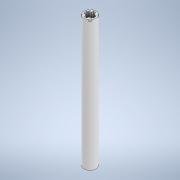
# Autodesk Inventor part: Upper Arm
Saved by Autodesk Inventor 2022 (Build 260153000, 153)
## iProperties
Created: 2022-03-03
Part Number: Upper Arm
Material: PLA Plastic
Document SubType Name: Modeling
Designer: Dahway
Density: 1.24912 g/cm^3
Appearance: PLA
Author: Dahway
Autodesk Inventor part; units mm, degrees
ref_plane "YZ Plane" through (0, 0, 0) normal (1, 0, 0) x (0, 1, 0)
ref_plane "XZ Plane" through (0, 0, 0) normal (0, 1, 0) x (-1, 0, 0)
ref_plane "XY Plane" through (0, 0, 0) normal (0, 0, 1) x (1, 0, 0)
sketch "Sketch1" plane through (0, 0, 0) normal (0, 1, 0) x (-1, 0, 0)
  circle A0 centre (0, 0) radius 7
  dimension "d0" = 14
  constraints: 1 centre point, 1 coincident
  measures "d0" diameter of A0
extrude "Extrusion1" add sketch "Sketch1" along normal blind 158
sketch "Sketch2" plane through (0, 158, 0) normal (0, 1, 0) x (1, 0, 0)
  circle A0 centre (0, 0) radius 3.75
  line L0 (-5.25, -1.5) -> (-2.25, -1.5)
  line L1 (-2.25, -1.5) -> (-2.25, 1.5)
  line L2 (-2.25, 1.5) -> (-5.25, 1.5)
  line L3 (-5.25, 1.5) -> (-5.25, -1.5)
  line L4 (-5.25, -1.5) -> (-2.25, 1.5) construction
  line L5 (-2.25, -1.5) -> (-5.25, 1.5) construction
  line L6 (-1.5, 2.25) -> (1.5, 2.25)
  line L7 (1.5, 2.25) -> (1.5, 5.25)
  line L8 (1.5, 5.25) -> (-1.5, 5.25)
  line L9 (-1.5, 5.25) -> (-1.5, 2.25)
  line L10 (-1.5, 2.25) -> (1.5, 5.25) construction
  line L11 (1.5, 2.25) -> (-1.5, 5.25) construction
  line L12 (2.25, 1.5) -> (5.25, 1.5)
  line L13 (5.25, 1.5) -> (5.25, -1.5)
  line L14 (5.25, -1.5) -> (2.25, -1.5)
  line L15 (2.25, -1.5) -> (2.25, 1.5)
  line L16 (2.25, 1.5) -> (5.25, -1.5) construction
  line L17 (5.25, 1.5) -> (2.25, -1.5) construction
  line L18 (-1.5, -5.25) -> (1.5, -5.25)
  line L19 (1.5, -5.25) -> (1.5, -2.25)
  line L20 (1.5, -2.25) -> (-1.5, -2.25)
  line L21 (-1.5, -2.25) -> (-1.5, -5.25)
  line L22 (-1.5, -5.25) -> (1.5, -2.25) construction
  line L23 (1.5, -5.25) -> (-1.5, -2.25) construction
  point P0 (-3.75, 0)
  point P1 (0, 3.75)
  point P2 (3.75, 0)
  point P3 (0, -3.75)
  point P4 (-3.4369, -1.5)
  point P5 (-1.5, -3.4369)
  point P6 (1.5, -3.4369)
  point P7 (3.4369, -1.5)
  point P8 (3.4369, 1.5)
  point P9 (1.5, 3.4369)
  point P10 (-1.5, 3.4369)
  point P11 (-3.4369, 1.5)
  dimension "d58" = 7.5
  dimension "d59" = 3
  dimension "d60" = 3
  dimension "d61" = 3
  dimension "d62" = 3
  dimension "d63" = 3
  dimension "d64" = 3
  dimension "d65" = 3
  dimension "d66" = 3
  constraints: 48 end point, 8 midpoint, 8 parallel, 4 horizontal, 4 perpendicular, 4 point on circle, 3 point on line, 1 centre point
  measures "d58" diameter of A0
  measures "d59" distance of L2.end L1.end
  measures "d60" distance of L1.end L0.end
  measures "d61" distance of L8.end L7.end
  measures "d62" distance of L7.end L6.end
  measures "d63" distance of L13.end L14.end
  measures "d64" distance of L12.end L13.end
  measures "d65" distance of L20.end L19.end
  measures "d66" distance of L19.end L18.end
extrude "Extrusion2" cut sketch "Sketch2" against normal through all
sketch "Sketch3" plane through (0, 158, 0) normal (0, 1, 0) x (1, 0, 0)
  circle A0 centre (0, 0) radius 9
  line L0 (-0.258, -9) -> (-0.258, -9)
  line L1 (-0.258, -11) -> (-0.258, -11)
  line L2 (-0.5, -9.5) -> (0.5, -9.5)
  line L3 (0.5, -9.5) -> (0.5, -8.5)
  line L4 (0.5, -8.5) -> (-0.5, -8.5)
  line L5 (-0.5, -8.5) -> (-0.5, -9.5)
  line L6 (-0.5, -9.5) -> (0.5, -8.5) construction
  line L7 (0.5, -9.5) -> (-0.5, -8.5) construction
  line L8 (-0.5, 8.5) -> (0.5, 8.5)
  line L9 (0.5, 8.5) -> (0.5, 9.5)
  line L10 (0.5, 9.5) -> (-0.5, 9.5)
  line L11 (-0.5, 9.5) -> (-0.5, 8.5)
  line L12 (-0.5, 8.5) -> (0.5, 9.5) construction
  line L13 (0.5, 8.5) -> (-0.5, 9.5) construction
  point P0 (0.492, 8.9865)
  point P1 (-0.258, -8.9963)
  point P2 (0, -9)
  point P3 (0, 9)
  point P4 (0.5, -8.9861)
  point P5 (-0.5, -8.9861)
  point P6 (-0.5, 8.9861)
  point P7 (0.5, 8.9861)
  dimension "d15" = 18
  dimension "d19" = 9
  dimension "d36" = 1
  dimension "d37" = 1
  dimension "d38" = 1
  dimension "d39" = 1
  constraints: 28 end point, 5 parallel, 4 midpoint, 4 point on circle, 3 horizontal, 2 perpendicular, 1 centre point, 1 coincident
  measures "d15" diameter of A0
  measures "d19" distance from line of A0.centre L0
  measures "d36" distance of L4.end L3.end
  measures "d37" distance of L3.end L2.end
  measures "d38" distance of L10.end L9.end
  measures "d39" distance of L9.end L8.end
extrude "Extrusion3" cut sketch "Sketch3" against normal blind 8
sketch "Sketch5" plane through (0, 0, 0) normal (0, -1, 0) x (1, 0, 0)
  line L0 (-1.25, 3.25) -> (-1.25, 1.25)
  line L1 (-1.25, 1.25) -> (-3.25, 1.25)
  line L2 (3.25, 1.25) -> (1.25, 1.25)
  line L3 (1.25, 1.25) -> (1.25, 3.25)
  line L4 (1.25, -3.25) -> (1.25, -1.25)
  line L5 (1.25, -1.25) -> (3.25, -1.25)
  line L6 (-3.25, -1.25) -> (-1.25, -1.25)
  line L7 (-1.25, -1.25) -> (-1.25, -3.25)
  circle A0 centre (0, 0) radius 3.75
  line L8 (-3.4369, -1.5) -> (-5.25, -1.5) projected
  line L9 (-2.25, 1.5) -> (-5.25, 1.5)
  line L10 (-5.25, 1.5) -> (-5.25, -1.5)
  line L11 (-5.25, -1.5) -> (-2.25, -1.5)
  line L12 (-2.25, -1.5) -> (-2.25, 1.5)
  line L13 (-2.25, 1.5) -> (-5.25, -1.5) construction
  line L14 (-5.25, 1.5) -> (-2.25, -1.5) construction
  line L15 (-1.5, -5.25) -> (-1.5, -3.4369) projected
  line L16 (1.5, -2.25) -> (-1.5, -2.25)
  line L17 (-1.5, -2.25) -> (-1.5, -5.25)
  line L18 (-1.5, -5.25) -> (1.5, -5.25)
  line L19 (1.5, -5.25) -> (1.5, -2.25)
  line L20 (1.5, -2.25) -> (-1.5, -5.25) construction
  line L21 (-1.5, -2.25) -> (1.5, -5.25) construction
  line L22 (1.5, 2.25) -> (-1.5, 2.25)
  line L23 (-1.5, 2.25) -> (-1.5, 5.25)
  line L24 (-1.5, 5.25) -> (1.5, 5.25)
  line L25 (1.5, 5.25) -> (1.5, 2.25)
  line L26 (1.5, 2.25) -> (-1.5, 5.25) construction
  line L27 (-1.5, 2.25) -> (1.5, 5.25) construction
  line L28 (5.25, 1.5) -> (5.25, -1.5) projected
  line L29 (2.25, 1.5) -> (5.25, 1.5)
  line L30 (5.25, 1.5) -> (5.25, -1.5)
  line L31 (5.25, -1.5) -> (2.25, -1.5)
  line L32 (2.25, -1.5) -> (2.25, 1.5)
  line L33 (2.25, 1.5) -> (5.25, -1.5) construction
  line L34 (5.25, 1.5) -> (2.25, -1.5) construction
  point P0 (-3.25, 3.25)
  point P1 (3.25, -3.25)
  point P2 (-3.75, 0)
  point P3 (0, -3.75)
  point P4 (0, 3.75)
  point P5 (3.75, 0)
  point P6 (3.4369, -1.5)
  point P7 (3.4369, 1.5)
  point P8 (-1.5, 3.4369)
  point P9 (1.5, 3.4369)
  point P10 (-3.4369, 1.5)
  point P11 (1.5, -3.4369)
  dimension "d54" = 360
  constraints: 66 end point, 8 midpoint, 8 parallel, 4 horizontal, 4 perpendicular, 4 point on circle, 4 point on line, 1 centre point, 1 coincident, 21 other
extrude "Extrusion5" add sketch "Sketch5" against normal blind 30 contours L23 L24 L25 A0 | A0 L8 L10 L9 | L29 L28 L31 A0 | A0 L19 L18 L15
sketch "Sketch6" plane through (0, 150, 0) normal (0, 1, 0) x (1, 0, 0)
  circle A0 centre (0, 0) radius 7 projected
  line L0 (0, 0) -> (7, 0) construction
  circle A1 centre (-4.9497, 4.9497) radius 1
  circle A2 centre (-4.9497, -4.9497) radius 1
  circle A3 centre (4.9497, -4.9497) radius 1
  circle A4 centre (4.9497, 4.9497) radius 1
  dimension "d69" = 2
  dimension "d70" = 4.9497
  dimension "d71" = 4.9497
  dimension "d74" = 360
  constraints: 4 centre point, 2 end point, 1 horizontal, 9 other
  measures "d69" diameter of A1
  measures "d70" horizontal distance of A0.centre A1.centre
  measures "d71" horizontal distance of A0.centre A1.centre
extrude "Extrusion6" cut sketch "Sketch6" against normal blind 2 contours A4 A0 | A0 A4 | A3 A0 | A0 A3 | A1 A0 | A0 A1 | A2 A0 | A0 A2
sketch "Sketch7" plane through (0, 150, 0) normal (0, 1, 0) x (1, 0, 0)
  line L0 (-4.75, 2.5) -> (4.75, 2.5)
  line L1 (4.75, 2.5) -> (4.75, -2.5)
  line L2 (4.75, -2.5) -> (-4.75, -2.5)
  line L3 (-4.75, -2.5) -> (-4.75, 2.5)
  line L4 (-4.75, 2.5) -> (4.75, -2.5) construction
  line L5 (4.75, 2.5) -> (-4.75, -2.5) construction
  point P0 (0, 0)
  dimension "d78" = 9.5
  dimension "d79" = 5
  constraints: 12 end point, 2 midpoint, 2 parallel, 1 horizontal, 1 perpendicular
  measures "d78" distance of L1.end L2.end
  measures "d79" distance of L0.end L1.end
extrude "Extrusion7" cut sketch "Sketch7" against normal through all
body "Solid1"
